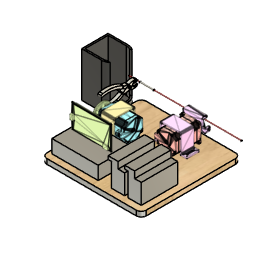
Full Project (Autodesk Fusion 360 design; units mm, degrees)
part number: 2025-08-30-11-35-49-750
Autodesk Fusion 360 part; units mm, degrees
note: some values were not read from the file. Set by a fixed rule: which sketch regions a step uses.
sketch "Sketch1" plane through (0, 0, 0) normal (0, 0, 1) x (1, 0, 0)
  line L0 (150, 150) -> (-150, 150)
  line L1 (-150, 150) -> (-150, -150)
  line L2 (-150, -150) -> (150, -150)
  line L3 (150, -150) -> (150, 150)
  line L4 (150, 150) -> (-150, -150) construction
  line L5 (-150, 150) -> (150, -150) construction
  dimension "d13" = 300
  constraint horizontal L0
  constraint perpendicular L0 L1
  constraint parallel L0 L2
  constraint parallel L1 L3
  constraint coincident L4 origin
  constraint coincident L5 origin
  measures "d13" distance of L1.end L2.end
extrude "Extrude1" add sketch "Sketch1" along normal blind 15 makes body 1
fillet "Fillet1" radius 15 1 edges at (150, -150, 7.5) on bodies 1
fillet "Fillet2" radius 15 1 edges at (-150, -150, 7.5) on bodies 1
fillet "Fillet3" radius 15 1 edges at (-150, 150, 7.5) on bodies 1
fillet "Fillet4" radius 15 1 edges at (150, 150, 7.5) on bodies 1
other "Base Mesh Feature1"
other "Base Mesh Feature2"
other "Modify1"
other "Base Mesh Feature3"
other "Modify2"
other "Modify3"
other "Modify4"
other "Modify5"
other "Base Mesh Feature4"
other "Base Mesh Feature5"
other "Modify6"
other "Modify7"
other "Modify8"
other "Modify9"
other "Modify10"
other "Modify11"
other "Modify12"
sketch "Sketch2" plane through (0, 0, 15) normal (0, 0, 1) x (-1, 0, 0)
  arc A0 (-150, -135) -> (-135, -150) centre (-135, -135) ccw
  line L0 (-135, -150) -> (135, -150)
  arc A1 (135, -150) -> (150, -135) centre (135, -135) ccw
  line L1 (150, -135) -> (150, 135)
  arc A2 (150, 135) -> (135, 150) centre (135, 135) ccw
  line L2 (135, 150) -> (-135, 150)
  arc A3 (-135, 150) -> (-150, 135) centre (-135, 135) ccw
  line L3 (-150, 135) -> (-150, -135)
  line L4 (-130, 130) -> (-90, 130)
  line L5 (-90, 130) -> (-90, 20)
  line L6 (-90, 20) -> (-130, 20)
  line L7 (-130, 20) -> (-130, 130)
  line L8 (-80, 130) -> (-40, 130)
  line L9 (-40, 130) -> (-40, 20)
  line L10 (-40, 20) -> (-80, 20)
  line L11 (-80, 20) -> (-80, 130)
  line L12 (10, 130) -> (140, 130)
  line L13 (140, 130) -> (140, 40)
  line L14 (140, 40) -> (10, 40)
  line L15 (10, 40) -> (10, 130)
  constraint horizontal L4
  constraint vertical L5
  constraint horizontal L6
  constraint vertical L7
  constraint horizontal L8
  constraint vertical L9
  constraint horizontal L10
  constraint vertical L11
  constraint horizontal L12
  constraint vertical L13
  constraint horizontal L14
  constraint vertical L15
extrude "Extrude2" add sketch "Sketch2" along normal blind 60 contours L4 L5 L6 L7 | L8 L9 L10 L11 bodies 1
sketch "Sketch3" plane through (0, 0, 75) normal (0, 0, 1) x (-1, 0, 0)
  line L0 (-130, 20) -> (-90, 20)
  line L1 (-90, 20) -> (-90, 130)
  line L2 (-90, 130) -> (-130, 130)
  line L3 (-130, 130) -> (-130, 20)
  line L4 (-110, 130) -> (-90, 130)
  line L5 (-90, 130) -> (-90, 20)
  line L6 (-90, 20) -> (-110, 20)
  line L7 (-110, 20) -> (-110, 130)
  line L8 (-60, 130) -> (-40, 130)
  line L9 (-40, 130) -> (-40, 20)
  line L10 (-40, 20) -> (-60, 20)
  line L11 (-60, 20) -> (-60, 130)
  constraint horizontal L4
  constraint vertical L5
  constraint horizontal L6
  constraint vertical L7
  constraint coincident L1 L0.end
  constraint horizontal L8
  constraint vertical L9
  constraint horizontal L10
  constraint vertical L11
extrude "Extrude3" add sketch "Sketch3" along normal blind 20 contours L0 L1 L2 L4 L5 L6 L7 | L8 L9 L10 L11 bodies 1
sketch "Sketch4" plane through (40, 0, 0) normal (-1, 0, 0) x (0, -1, 0)
  line L0 (20, 15) -> (130, 15)
  line L1 (130, 15) -> (130, 95)
  line L2 (130, 95) -> (20, 95)
  line L3 (20, 95) -> (20, 15)
  line L4 (20, 95) -> (130, 95)
  line L5 (130, 95) -> (130, 85)
  line L6 (130, 85) -> (20, 85)
  line L7 (20, 85) -> (20, 95)
  constraint horizontal L4
  constraint vertical L5
  constraint horizontal L6
  constraint vertical L7
  constraint coincident L2.end L3.start
sketch "Sketch5" plane through (90, 0, 0) normal (-1, 0, 0) x (0, -1, 0)
  line L0 (20, 15) -> (130, 15)
  line L1 (130, 15) -> (130, 95)
  line L2 (130, 95) -> (20, 95)
  line L3 (20, 95) -> (20, 15)
  line L4 (20, 95) -> (130, 95)
  line L5 (130, 95) -> (130, 85)
  line L6 (130, 85) -> (20, 85)
  line L7 (20, 85) -> (20, 95)
  constraint horizontal L4
  constraint vertical L5
  constraint horizontal L6
  constraint vertical L7
  constraint coincident L2.end L3.start
extrude "Extrude4" add sketch "Sketch5" along normal blind 10 contours L1 L2 L3 L4 L5 L6 L7 bodies 1
extrude "Extrude5" add sketch "Sketch4" along normal blind 10 contours L1 L2 L3 L4 L5 L6 L7 bodies 1
sketch "Sketch6" plane through (0, 0, 15) normal (0, 0, 1) x (-1, 0, 0)
  line L0 (-80, 20) -> (-80, 130)
  line L1 (-80, 130) -> (-40, 130)
  line L2 (-40, 130) -> (-40, 20)
  line L3 (-40, 20) -> (-80, 20)
  line L4 (-130, 20) -> (-130, 130)
  line L5 (-130, 130) -> (-90, 130)
  line L6 (-90, 130) -> (-90, 20)
  line L7 (-90, 20) -> (-130, 20)
  arc A0 (-150, -135) -> (-135, -150) centre (-135, -135) ccw
  line L8 (-135, -150) -> (135, -150)
  arc A1 (135, -150) -> (150, -135) centre (135, -135) ccw
  line L9 (150, -135) -> (150, 135)
  arc A2 (150, 135) -> (135, 150) centre (135, 135) ccw
  line L10 (135, 150) -> (-135, 150)
  arc A3 (-135, 150) -> (-150, 135) centre (-135, 135) ccw
  line L11 (-150, 135) -> (-150, -135)
  line L12 (0, 130) -> (140, 130)
  line L13 (140, 130) -> (140, 30)
  line L14 (140, 30) -> (0, 30)
  line L15 (0, 30) -> (0, 130)
  constraint horizontal L12
  constraint vertical L13
  constraint horizontal L14
  constraint vertical L15
extrude "Extrude6" add sketch "Sketch6" along normal blind 40 contours L12 L13 L14 L15 bodies 1
other "Base Mesh Feature7"
other "Modify13"
other "Base Mesh Feature8"
sketch "Sketch7" plane through (0, 0, 15) normal (0, 0, 1) x (-1, 0, 0)
  line L0 (0, 30) -> (0, 130)
  line L1 (0, 130) -> (140, 130)
  line L2 (140, 130) -> (140, 30)
  line L3 (140, 30) -> (0, 30)
  line L4 (-80, 20) -> (-80, 130)
  line L5 (-80, 130) -> (-40, 130)
  line L6 (-40, 130) -> (-40, 20)
  line L7 (-40, 20) -> (-80, 20)
  line L8 (-130, 20) -> (-130, 130)
  line L9 (-130, 130) -> (-90, 130)
  line L10 (-90, 130) -> (-90, 20)
  line L11 (-90, 20) -> (-130, 20)
  arc A0 (-150, -135) -> (-135, -150) centre (-135, -135) ccw
  line L12 (-135, -150) -> (135, -150)
  arc A1 (135, -150) -> (150, -135) centre (135, -135) ccw
  line L13 (150, -135) -> (150, 135)
  arc A2 (150, 135) -> (135, 150) centre (135, 135) ccw
  line L14 (135, 150) -> (-135, 150)
  arc A3 (-135, 150) -> (-150, 135) centre (-135, 135) ccw
  line L15 (-150, 135) -> (-150, -135)
  line L16 (190, -70) -> (250, -70)
  line L17 (250, -70) -> (250, -150)
  line L18 (250, -150) -> (190, -150)
  line L19 (160, -120) -> (160, -100)
  arc A4 (190, -70) -> (160, -100) centre (190, -100) ccw
  arc A5 (160, -120) -> (190, -150) centre (190, -120) ccw
  dimension "d24" = 30
  constraint horizontal L16
  constraint vertical L17
  constraint horizontal L18
  constraint vertical L19
  constraint tangent L16 A4
  constraint tangent L19 A4
  constraint tangent L18 A5
  constraint tangent L19 A5
  constraint equal A4 A5
  measures "d24" radius of A4
extrude "Extrude7" add sketch "Sketch7" along normal blind 120 separate body contours L16 L17 L18 L19 A4 A5 makes body 2
extrude "Extrude8" add 1 faces at (-230, 123.3333, 15) along direction (0, 0, -1) blind 15 on bodies 2 bodies 2
shell "Shell1" thickness 5 removed faces 1 at (-230, 123.3333, 135) on bodies 2
ref_plane "WorkPlane1" through (-160.005, 120.5456, 96.719) normal (0.999835, 0.018187, 0) x (0.018187, -0.999835, 0)
sketch "Sketch8" plane through (-157.76, -2.8697, 0) normal (0.999835, 0.018187, 0) x (0.018187, -0.999835, 0)
  line L0 (-80, -135) -> (-145, -135)
  line L1 (-145, -135) -> (-145, -15)
  line L2 (-145, -15) -> (-80, -15)
  line L3 (-80, -15) -> (-80, -135)
  constraint horizontal L0
  constraint vertical L1
  constraint horizontal L2
  constraint vertical L3
extrude "Extrude9" cut sketch "Sketch8" against normal blind 30 bodies 2
ref_plane "WorkPlane2" through (-142, 0, 0) normal (1, 0, 0) x (0, 1, 0)
sketch "Sketch9" plane through (-142, 0, 0) normal (1, 0, 0) x (0, 1, 0)
  spline S0 degree 3 poles (163.1684, -45.0756) (99.6684, -45.0756) (36.1684, -45.0756) (-27.3316, -45.0756) knots 0 0 0 0 1 1 1 1
  spline S1 degree 3 poles (-27.3316, -45.0756) (-27.3316, 18.4244) (-27.3316, 81.9244) (-27.3316, 145.4244) knots 0 0 0 0 1 1 1 1
  spline S2 degree 3 poles (-27.3316, 145.4244) (36.1684, 145.4244) (99.6684, 145.4244) (163.1684, 145.4244) knots 0 0 0 0 1 1 1 1
  spline S3 degree 3 poles (163.1684, 145.4244) (163.1684, 81.9244) (163.1684, 18.4244) (163.1684, -45.0756) knots 0 0 0 0 1 1 1 1
  spline S4 degree 3 poles (35.11, 32.7119) (37.7104, 32.6389) (40.18, 32.9913) (42.5184, 33.7702) knots 0 0 0 0 1 1 1 1
  spline S5 degree 3 poles (42.5184, 33.7702) (53.8679, 35.0842) (64.4513, 38.6116) (74.2684, 44.3536) knots 0 0 0 0 1 1 1 1
  spline S6 degree 3 poles (74.2684, 44.3536) (75.0775, 44.3382) (75.695, 43.9853) (76.1205, 43.2952) knots 0 0 0 0 1 1 1 1
  spline S7 degree 3 poles (76.1205, 43.2952) (77.2169, 41.4791) (77.5693, 39.5392) (77.1788, 37.4744) knots 0 0 0 0 1 1 1 1
  spline S8 degree 3 poles (77.1788, 37.4744) (57.7383, 26.6937) (37.0129, 23.0774) (15.0017, 26.6265) knots 0 0 0 0 1 1 1 1
  spline S9 degree 3 poles (15.0017, 26.6265) (10.408, 28.0939) (9.7021, 30.563) (12.885, 34.0348) knots 0 0 0 0 1 1 1 1
  spline S10 degree 3 poles (12.885, 34.0348) (20.2288, 32.9786) (27.6372, 32.5378) (35.11, 32.7119) knots 0 0 0 0 1 1 1 1
  spline S11 degree 3 poles (35.11, 32.7119) (37.4484, 33.4908) (39.9181, 33.8433) (42.5184, 33.7702) knots 0 0 0 0 1 1 1 1
  spline S12 degree 3 poles (42.5184, 33.7702) (40.18, 32.9913) (37.7104, 32.6389) (35.11, 32.7119) knots 0 0 0 0 1 1 1 1
  spline S13 degree 3 poles (80.0892, 40.1202) (79.3235, 39.3873) (78.7943, 39.5636) (78.5017, 40.6494) knots 0 0 0 0 1 1 1 1
  spline S14 degree 3 poles (78.5017, 40.6494) (78.9732, 40.3266) (79.5024, 40.1504) (80.0892, 40.1202) knots 0 0 0 0 1 1 1 1
  spline S15 degree 3 poles (80.0892, 40.1202) (79.5024, 40.1504) (78.9732, 40.3266) (78.5017, 40.6494) knots 0 0 0 0 1 1 1 1
  spline S16 degree 3 poles (78.5017, 40.6494) (77.881, 42.0506) (77.4402, 43.4619) (77.1788, 44.8827) knots 0 0 0 0 1 1 1 1
  spline S17 degree 3 poles (77.1788, 44.8827) (79.7373, 46.4644) (82.1186, 48.2281) (84.3225, 50.1744) knots 0 0 0 0 1 1 1 1
  spline S18 degree 3 poles (84.3225, 50.1744) (87.9992, 52.4419) (91.5272, 54.911) (94.9059, 57.5827) knots 0 0 0 0 1 1 1 1
  spline S19 degree 3 poles (94.9059, 57.5827) (101.3755, 60.8138) (108.2546, 61.9605) (115.5434, 61.0223) knots 0 0 0 0 1 1 1 1
  spline S20 degree 3 poles (115.5434, 61.0223) (116.6761, 60.7191) (117.7345, 60.2783) (118.7184, 59.6994) knots 0 0 0 0 1 1 1 1
  spline S21 degree 3 poles (118.7184, 59.6994) (116.9545, 59.3464) (115.1906, 58.994) (113.4267, 58.6411) knots 0 0 0 0 1 1 1 1
  spline S22 degree 3 poles (113.4267, 58.6411) (112.5383, 58.4336) (111.6564, 58.1691) (110.7809, 57.8473) knots 0 0 0 0 1 1 1 1
  spline S23 degree 3 poles (110.7809, 57.8473) (109.0786, 56.9398) (107.844, 55.6169) (107.0767, 53.8786) knots 0 0 0 0 1 1 1 1
  spline S24 degree 3 poles (107.0767, 53.8786) (104.9415, 50.0675) (102.119, 46.8041) (98.61, 44.089) knots 0 0 0 0 1 1 1 1
  spline S25 degree 3 poles (98.61, 44.089) (96.9077, 43.2227) (95.144, 42.5174) (93.3184, 41.9723) knots 0 0 0 0 1 1 1 1
  spline S26 degree 3 poles (93.3184, 41.9723) (88.8908, 41.4241) (84.4808, 40.8066) (80.0892, 40.1202) knots 0 0 0 0 1 1 1 1
  spline S27 degree 3 poles (107.0767, 47.5286) (108.4282, 45.5606) (110.1922, 44.0615) (112.3684, 43.0307) knots 0 0 0 0 1 1 1 1
  spline S28 degree 3 poles (112.3684, 43.0307) (115.3045, 42.8687) (118.1267, 42.7804) (120.835, 42.7661) knots 0 0 0 0 1 1 1 1
  spline S29 degree 3 poles (120.835, 42.7661) (113.3447, 39.4) (105.7602, 39.3122) (98.0809, 42.5015) knots 0 0 0 0 1 1 1 1
  spline S30 degree 3 poles (98.0809, 42.5015) (100.8781, 44.0641) (103.1715, 46.1808) (104.96, 48.8515) knots 0 0 0 0 1 1 1 1
  spline S31 degree 3 poles (104.96, 48.8515) (105.313, 49.2044) (105.6654, 49.2044) (106.0184, 48.8515) knots 0 0 0 0 1 1 1 1
  spline S32 degree 3 poles (106.0184, 48.8515) (106.3179, 48.325) (106.6708, 47.8842) (107.0767, 47.5286) knots 0 0 0 0 1 1 1 1
  spline S33 degree 3 poles (109.1934, 48.0577) (113.0582, 47.4423) (116.9387, 46.9132) (120.835, 46.4702) knots 0 0 0 0 1 1 1 1
  spline S34 degree 3 poles (120.835, 46.4702) (121.3642, 46.1173) (121.8934, 45.7649) (122.4225, 45.4119) knots 0 0 0 0 1 1 1 1
  spline S35 degree 3 poles (122.4225, 45.4119) (117.0609, 42.6459) (112.2984, 43.4397) (108.135, 47.7932) knots 0 0 0 0 1 1 1 1
  spline S36 degree 3 poles (108.135, 47.7932) (108.4494, 48.0387) (108.8023, 48.1271) (109.1934, 48.0577) knots 0 0 0 0 1 1 1 1
  spline S37 degree 3 poles (120.835, 42.7661) (118.1267, 42.7804) (115.3045, 42.8687) (112.3684, 43.0307) knots 0 0 0 0 1 1 1 1
  spline S38 degree 3 poles (112.3684, 43.0307) (110.1922, 44.0615) (108.4282, 45.5606) (107.0767, 47.5286) knots 0 0 0 0 1 1 1 1
  spline S39 degree 3 poles (107.0767, 47.5286) (107.4238, 47.9403) (107.8646, 48.2927) (108.3996, 48.5869) knots 0 0 0 0 1 1 1 1
  spline S40 degree 3 poles (108.3996, 48.5869) (108.8044, 48.5499) (109.069, 48.3736) (109.1934, 48.0577) knots 0 0 0 0 1 1 1 1
  spline S41 degree 3 poles (109.1934, 48.0577) (108.8023, 48.1271) (108.4494, 48.0387) (108.135, 47.7932) knots 0 0 0 0 1 1 1 1
  spline S42 degree 3 poles (108.135, 47.7932) (112.2984, 43.4397) (117.0609, 42.6459) (122.4225, 45.4119) knots 0 0 0 0 1 1 1 1
  spline S43 degree 3 poles (122.4225, 45.4119) (122.6435, 45.0298) (122.9963, 44.7653) (123.4809, 44.6182) knots 0 0 0 0 1 1 1 1
  spline S44 degree 3 poles (123.4809, 44.6182) (122.7685, 43.735) (121.8865, 43.1174) (120.835, 42.7661) knots 0 0 0 0 1 1 1 1
  spline S45 degree 3 poles (122.4225, 45.4119) (121.8934, 45.7649) (121.3642, 46.1173) (120.835, 46.4702) knots 0 0 0 0 1 1 1 1
  spline S46 degree 3 poles (120.835, 46.4702) (121.6171, 46.6089) (122.3226, 46.4327) (122.9517, 45.9411) knots 0 0 0 0 1 1 1 1
  spline S47 degree 3 poles (122.9517, 45.9411) (122.8863, 45.6199) (122.7099, 45.4437) (122.4225, 45.4119) knots 0 0 0 0 1 1 1 1
  spline S48 degree 3 poles (83.7934, 51.2327) (81.6582, 53.0091) (79.3653, 54.5966) (76.9142, 55.9952) knots 0 0 0 0 1 1 1 1
  spline S49 degree 3 poles (76.9142, 55.9952) (77.5953, 57.533) (78.1244, 59.1205) (78.5017, 60.7577) knots 0 0 0 0 1 1 1 1
  spline S50 degree 3 poles (78.5017, 60.7577) (79.0309, 60.7577) (79.56, 60.7577) (80.0892, 60.7577) knots 0 0 0 0 1 1 1 1
  spline S51 degree 3 poles (80.0892, 60.7577) (83.9447, 60.145) (87.8256, 59.7036) (91.7309, 59.4348) knots 0 0 0 0 1 1 1 1
  spline S52 degree 3 poles (91.7309, 59.4348) (92.9183, 59.4084) (93.8005, 58.9676) (94.3767, 58.1119) knots 0 0 0 0 1 1 1 1
  spline S53 degree 3 poles (94.3767, 58.1119) (90.8488, 55.819) (87.3213, 53.5256) (83.7934, 51.2327) knots 0 0 0 0 1 1 1 1
  spline S54 degree 3 poles (84.3225, 50.1744) (84.1463, 50.5274) (83.9696, 50.8798) (83.7934, 51.2327) knots 0 0 0 0 1 1 1 1
  spline S55 degree 3 poles (83.7934, 51.2327) (87.3213, 53.5256) (90.8488, 55.819) (94.3767, 58.1119) knots 0 0 0 0 1 1 1 1
  spline S56 degree 3 poles (94.3767, 58.1119) (94.3767, 57.7589) (94.5529, 57.5827) (94.9059, 57.5827) knots 0 0 0 0 1 1 1 1
  spline S57 degree 3 poles (94.9059, 57.5827) (91.5272, 54.911) (87.9992, 52.4419) (84.3225, 50.1744) knots 0 0 0 0 1 1 1 1
  spline S58 degree 3 poles (97.5517, 46.4702) (92.1918, 46.7909) (90.9567, 49.1722) (93.8475, 53.614) knots 0 0 0 0 1 1 1 1
  spline S59 degree 3 poles (93.8475, 53.614) (98.1386, 55.1311) (100.1669, 53.632) (99.933, 49.1161) knots 0 0 0 0 1 1 1 1
  spline S60 degree 3 poles (99.933, 49.1161) (99.2101, 48.1308) (98.4164, 47.2492) (97.5517, 46.4702) knots 0 0 0 0 1 1 1 1
  spline S61 degree 3 poles (97.5517, 48.0577) (93.1189, 47.9381) (92.2368, 49.614) (94.9059, 53.0848) knots 0 0 0 0 1 1 1 1
  spline S62 degree 3 poles (94.9059, 53.0848) (98.6116, 52.9822) (99.4932, 51.3068) (97.5517, 48.0577) knots 0 0 0 0 1 1 1 1
  spline S63 degree 3 poles (109.1934, 53.3494) (108.0578, 53.4531) (107.97, 53.9823) (108.9288, 54.9369) knots 0 0 0 0 1 1 1 1
  spline S64 degree 3 poles (108.9288, 54.9369) (110.0292, 55.7957) (111.1757, 56.5895) (112.3684, 57.3182) knots 0 0 0 0 1 1 1 1
  spline S65 degree 3 poles (112.3684, 57.3182) (115.0142, 57.6711) (117.66, 57.6711) (120.3059, 57.3182) knots 0 0 0 0 1 1 1 1
  spline S66 degree 3 poles (120.3059, 57.3182) (121.3877, 57.0546) (122.0933, 56.4371) (122.4225, 55.4661) knots 0 0 0 0 1 1 1 1
  spline S67 degree 3 poles (122.4225, 55.4661) (117.9974, 54.8448) (113.5877, 54.1389) (109.1934, 53.3494) knots 0 0 0 0 1 1 1 1
  spline S68 degree 3 poles (48.3392, 65.5202) (46.5009, 66.0626) (44.561, 66.4156) (42.5184, 66.5786) knots 0 0 0 0 1 1 1 1
  spline S69 degree 3 poles (42.5184, 66.5786) (33.14, 67.7163) (23.8796, 67.1871) (14.7371, 64.9911) knots 0 0 0 0 1 1 1 1
  spline S70 degree 3 poles (14.7371, 64.9911) (11.0049, 65.2588) (9.7704, 67.1988) (11.033, 70.8119) knots 0 0 0 0 1 1 1 1
  spline S71 degree 3 poles (11.033, 70.8119) (12.4998, 72.0084) (14.1752, 72.8021) (16.06, 73.1932) knots 0 0 0 0 1 1 1 1
  spline S72 degree 3 poles (16.06, 73.1932) (37.2087, 76.6788) (57.3171, 73.5038) (76.385, 63.6682) knots 0 0 0 0 1 1 1 1
  spline S73 degree 3 poles (76.385, 63.6682) (76.8512, 63.2935) (77.2037, 62.8522) (77.4434, 62.3452) knots 0 0 0 0 1 1 1 1
  spline S74 degree 3 poles (77.4434, 62.3452) (77.219, 60.4868) (76.6899, 58.7231) (75.8559, 57.0536) knots 0 0 0 0 1 1 1 1
  spline S75 degree 3 poles (75.8559, 57.0536) (75.0262, 56.5387) (74.144, 56.4503) (73.21, 56.789) knots 0 0 0 0 1 1 1 1
  spline S76 degree 3 poles (73.21, 56.789) (65.3937, 61.0795) (57.1033, 63.9899) (48.3392, 65.5202) knots 0 0 0 0 1 1 1 1
  spline S77 degree 3 poles (109.1934, 53.3494) (109.069, 53.0335) (108.8044, 52.8573) (108.3996, 52.8202) knots 0 0 0 0 1 1 1 1
  spline S78 degree 3 poles (108.3996, 52.8202) (107.8646, 53.1145) (107.4238, 53.4669) (107.0767, 53.8786) knots 0 0 0 0 1 1 1 1
  spline S79 degree 3 poles (107.0767, 53.8786) (107.844, 55.6169) (109.0786, 56.9398) (110.7809, 57.8473) knots 0 0 0 0 1 1 1 1
  spline S80 degree 3 poles (110.7809, 57.8473) (111.6564, 58.1691) (112.5383, 58.4336) (113.4267, 58.6411) knots 0 0 0 0 1 1 1 1
  spline S81 degree 3 poles (113.4267, 58.6411) (116.3521, 58.9057) (119.1744, 58.5527) (121.8934, 57.5827) knots 0 0 0 0 1 1 1 1
  spline S82 degree 3 poles (121.8934, 57.5827) (122.2144, 57.6484) (122.3908, 57.8246) (122.4225, 58.1119) knots 0 0 0 0 1 1 1 1
  spline S83 degree 3 poles (122.4225, 58.1119) (123.7044, 57.2928) (123.7044, 56.4112) (122.4225, 55.4661) knots 0 0 0 0 1 1 1 1
  spline S84 degree 3 poles (122.4225, 55.4661) (122.0933, 56.4371) (121.3877, 57.0546) (120.3059, 57.3182) knots 0 0 0 0 1 1 1 1
  spline S85 degree 3 poles (120.3059, 57.3182) (117.66, 57.6711) (115.0142, 57.6711) (112.3684, 57.3182) knots 0 0 0 0 1 1 1 1
  spline S86 degree 3 poles (112.3684, 57.3182) (111.1757, 56.5895) (110.0292, 55.7957) (108.9288, 54.9369) knots 0 0 0 0 1 1 1 1
  spline S87 degree 3 poles (108.9288, 54.9369) (107.97, 53.9823) (108.0578, 53.4531) (109.1934, 53.3494) knots 0 0 0 0 1 1 1 1
  spline S88 degree 3 poles (122.4225, 58.1119) (122.3908, 57.8246) (122.2144, 57.6484) (121.8934, 57.5827) knots 0 0 0 0 1 1 1 1
  spline S89 degree 3 poles (121.8934, 57.5827) (119.1744, 58.5527) (116.3521, 58.9057) (113.4267, 58.6411) knots 0 0 0 0 1 1 1 1
  spline S90 degree 3 poles (113.4267, 58.6411) (115.1906, 58.994) (116.9545, 59.3464) (118.7184, 59.6994) knots 0 0 0 0 1 1 1 1
  spline S91 degree 3 poles (118.7184, 59.6994) (119.9965, 59.2734) (121.2312, 58.7443) (122.4225, 58.1119) knots 0 0 0 0 1 1 1 1
  spline S92 degree 3 poles (76.9142, 55.9952) (76.5613, 56.3482) (76.2088, 56.7006) (75.8559, 57.0536) knots 0 0 0 0 1 1 1 1
  spline S93 degree 3 poles (75.8559, 57.0536) (76.6899, 58.7231) (77.219, 60.4868) (77.4434, 62.3452) knots 0 0 0 0 1 1 1 1
  spline S94 degree 3 poles (77.4434, 62.3452) (78.2578, 61.6748) (79.1399, 61.1456) (80.0892, 60.7577) knots 0 0 0 0 1 1 1 1
  spline S95 degree 3 poles (80.0892, 60.7577) (79.56, 60.7577) (79.0309, 60.7577) (78.5017, 60.7577) knots 0 0 0 0 1 1 1 1
  spline S96 degree 3 poles (78.5017, 60.7577) (78.1244, 59.1205) (77.5953, 57.533) (76.9142, 55.9952) knots 0 0 0 0 1 1 1 1
  spline S97 degree 3 poles (48.3392, 65.5202) (46.2284, 65.317) (44.2884, 65.67) (42.5184, 66.5786) knots 0 0 0 0 1 1 1 1
  spline S98 degree 3 poles (42.5184, 66.5786) (44.561, 66.4156) (46.5009, 66.0626) (48.3392, 65.5202) knots 0 0 0 0 1 1 1 1
other "Modify14"
extrude "Extrude10" add sketch "Sketch9" against normal blind 10 separate body contours S4 S5 S6 S7 S8 S9 S10 S12 | S14 S15 S16 S17 S18 S19 S20 S21 S22 S23 S24 S25 S26 S57 S79 S80 S90 | S48 S49 S50 S51 S52 S53 S55 S95 S96 | S63 S64 S65 S66 S67 S84 S85 S86 S87 | S68 S69 S70 S71 S72 S73 S74 S75 S76 S93 S98 | S27 S28 S29 S30 S31 S32 S37 S38 | S33 S34 S35 S36 S41 S42 S45 | S61 S62 makes body 3 at (-145.3333, 72.9067, 35.2309) makes body 4 at (-148.6667, 87.3212, 53.5258) makes body 5 at (-142, 84.7637, 43.1615) makes body 6 at (-147.5556, 101.9444, 41.1713) makes body 7 at (-146.4444, 120.9481, 55.2559) makes body 8 at (-146.4444, 47.836, 73.2906) makes body 9 at (-147.5556, 120.6575, 44.6218) makes body 10 at (-147.5556, 96.8458, 48.0544)
move_body "Move1" bodies 10 8 4 3 9 5 7 6 to x (1, 0, 0) y (0, 1, 0) z (0, 0, 1) at (0, 10, 20)
sketch "Sketch10" plane through (0, 0, 0) normal (1, 0, 0) x (0, 1, 0)
  circle A0 centre (133.2974, 72.7966) radius 2
  dimension "d36" = 4
  measures "d36" diameter of A0
extrude "Extrude11" add sketch "Sketch10" along normal mid plane 340 separate body makes body 11
other "Base Mesh Feature9"
other "Modify15"
ref_plane "WorkPlane3" through (-125, 0, 0) normal (1, 0, 0) x (0, 1, 0)
sketch "Sketch11" plane through (-125, 0, 0) normal (1, 0, 0) x (0, 1, 0)
  circle A0 centre (133.3, 72.8) radius 2.3921
extrude "Extrude12" add sketch "Sketch11" against normal blind 12 bodies 11
extrude "Extrude13" add 1 faces at (-125, 134.0114, 74.9391) along direction (1, 0, 0) blind 30 on bodies 11 bodies 11
